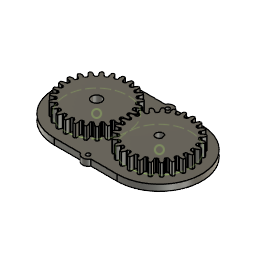
encoder gear system enclosed (Autodesk Fusion 360 design; units mm, degrees)
description: Spur Gear; Module: 2.0; Num Teeth: 25; Pressure Angle: 14.500000000000002; Backlash: 0.15 mm
Autodesk Fusion 360 part; units mm, degrees
(part 1 of 3)
sketch "Sketch1" plane through (0, 0, 0) normal (0, 0, 1) x (1, 0, 0) in component "casing bottom"
  circle A0 centre (0, 0) radius 19.5 construction
  circle A1 centre (50.4, 0) radius 15 construction
  circle A2 centre (0, 0) radius 15.5
  circle A3 centre (50.4, 0) radius 11
  circle A4 centre (13.7886, 13.7886) radius 2.2
  circle A5 centre (13.7886, 13.7886) radius 5.2
  circle A6 centre (-13.7886, 13.7886) radius 2.2
  circle A7 centre (-13.7886, 13.7886) radius 5.2
  circle A8 centre (-13.7886, -13.7886) radius 2.2
  circle A9 centre (-13.7886, -13.7886) radius 5.2
  circle A10 centre (13.7886, -13.7886) radius 2.2
  circle A11 centre (13.7886, -13.7886) radius 5.2
  line L0 (0, 0) -> (13.7886, 13.7886) construction
  line L1 (0, 0) -> (19.5, 0) construction
  circle A12 centre (35.4, 0) radius 1.7
  circle A13 centre (57.9, -12.9904) radius 1.7
  circle A14 centre (57.9, 12.9904) radius 1.7
  circle A15 centre (35.4, 0) radius 4.7
  circle A16 centre (57.9, -12.9904) radius 4.7
  circle A17 centre (57.9, 12.9904) radius 4.7
  circle A18 centre (0, 0) radius 30
  circle A19 centre (0, 0) radius 34
  line L2 (0, 0) -> (-30, 0) construction
  line L3 (50.4, 0) -> (80.4, 0) construction
  line L4 (80.4, 0) -> (84.4, 0) construction
  line L5 (-30, 0) -> (-34, 0) construction
  line L6 (0, 0) -> (50.4, 0) construction
  line L7 (25.2, 0) -> (25.2, 30) construction
  circle A20 centre (50.4, 0) radius 34
  circle A21 centre (50.4, 0) radius 30
  line L8 (0, 30) -> (50.4, 30)
  line L9 (0, 34) -> (50.4, 34)
  line L10 (0, -34) -> (50.4, -34)
  line L11 (0, -30) -> (50.4, -30)
  line L12 (25.2, 30) -> (25.2, 34) construction
  circle A22 centre (25.2, 32) radius 1.6
  circle A23 centre (25.2, 32) radius 4.6
  circle A24 centre (25.2, -32) radius 4.6
  circle A25 centre (25.2, -32) radius 1.6
  dimension "d189_1_1_1" = 39
  dimension "d190_1_1_1" = 30
  dimension "d191_1_1_1" = 50.4
  dimension "d193_1_1_1" = -4
  dimension "d195_1_1_1" = -4
  dimension "d196_1_1_1" = 4.4
  dimension "d197_1_1_1" = 3
  dimension "d199_1_1_1" = 360
  dimension "d200_1_1_1" = 45
  dimension "d201_1_1_1" = 3.4
  dimension "d209_1_1_1" = 3
  dimension "d211_1_1_1" = 360
  dimension "d243" = 60
  dimension "d245" = 4
  dimension "d261" = -4
  dimension "d264" = 3.2
  dimension "d268" = 3
  constraint coincident A0.centre A2.centre
  constraint coincident A0 A4.centre
  constraint horizontal A1.centre A0.centre
  constraint coincident A4.centre A5.centre
  constraint coincident A0 L1.end
  constraint horizontal L1
  constraint coincident A1 A12.centre
  constraint horizontal A1.centre A12.centre
  constraint coincident A19 L5.end
  constraint horizontal L2
  constraint coincident A1.centre A3.centre
  constraint parallel L2 L3
  constraint parallel L2 L4
  constraint coincident A18 L2.end
  constraint horizontal L5
  constraint midpoint L6 L7.start
  constraint perpendicular L6 L7
  constraint symmetric A18 L7 A21
  constraint symmetric A19 L7 A20
  constraint coincident A18 L8.start
  constraint coincident A21 L8.end
  constraint tangent A21 L8
  constraint tangent A18 L8
  constraint symmetric L6 L8.start L11.start
  constraint symmetric L6 L8.end L11.end
  constraint symmetric L6 L9.start L10.start
  constraint symmetric L6 L9.end L10.end
  constraint midpoint L12.end L9
  constraint coincident L8 L7.end
  constraint perpendicular L6 L12
  constraint symmetric A18 A21 L12
  constraint symmetric A19 A20 L12
  constraint midpoint L12 A22.centre
  constraint symmetric L6 A22 A25
  constraint symmetric L6 A23 A24
  measures "d189_1_1_1" diameter of A0
  measures "d190_1_1_1" diameter of A1
  measures "d191_1_1_1" distance of A0.centre A1.centre
  measures "d196_1_1_1" diameter of A4
  measures "d200_1_1_1" angle of L0 L1
  measures "d201_1_1_1" diameter of A12
  measures "d243" diameter of A18
  measures "d264" diameter of A22
extrude "Extrude5" add sketch "Sketch1" against normal blind 5 contours A2 A5 A7 A9 A11 | A2 A5 A11 A20 | A2 A5 | A2 A5 A20 | A2 A11 A20 | A2 A11 | A2 A5 A7 A9 A11 A18 A20 | A5 A20 | A5 A11 A18 A20 A21 | A11 A20 | A2 A7 | A2 A7 | A2 A9 | A2 A9 | A18 A19 A20 A21 | A18 A19 A20 L8 | A18 A19 A20 L11 | A18 A19 A20 A21 | A15 A18 A19 A21 | A18 A21 | A18 A19 L8 L11 | A19 A20 A21 L8 | A19 A20 L8 A23 | A19 A20 L11 A24 | A19 A20 A21 L11 | A3 A15 A16 A17 A19 A21 | A19 L8 L9 A23 | A20 L8 L9 A23 | A20 A21 L8 L11 | A19 L10 L11 A24 | A20 L10 L11 A24 | A12 A15 A19 | A3 A12 A15 A19 | L8 L9 A23 | L8 A23 | L11 A24 | L10 L11 A24 | L9 A23 | L10 A24 | A3 A17 | A3 A16 picked at (56.2758, 10.1772) picked at (56.2758, -10.1772) makes body 1 in component "casing bottom"
extrude "Extrude6" cut sketch "Sketch1" against normal blind 3 contours A12 A15 A19 | A3 A12 A15 A19 | A3 A17 | A3 A16 picked at (56.2758, 10.1772) picked at (56.2758, -10.1772) bodies 1 in component "casing bottom"
extrude "Extrude7" cut sketch "Sketch1" against normal blind 5 contours A2 A5 A7 A9 A11 bodies 1 in component "casing bottom"
sketch "Sketch1 (2)" plane through (0, 0, 0) normal (0, 0, 1) x (1, 0, 0) in component "casing top"
  circle A0 centre (0, 0) radius 19.5 construction
  circle A1 centre (50.4, 0) radius 15 construction
  circle A2 centre (0, 0) radius 15.5
  circle A3 centre (50.4, 0) radius 11
  circle A4 centre (13.7886, 13.7886) radius 2.2
  circle A5 centre (13.7886, 13.7886) radius 5.2
  circle A6 centre (-13.7886, 13.7886) radius 2.2
  circle A7 centre (-13.7886, 13.7886) radius 5.2
  circle A8 centre (-13.7886, -13.7886) radius 2.2
  circle A9 centre (-13.7886, -13.7886) radius 5.2
  circle A10 centre (13.7886, -13.7886) radius 2.2
  circle A11 centre (13.7886, -13.7886) radius 5.2
  line L0 (0, 0) -> (13.7886, 13.7886) construction
  line L1 (0, 0) -> (19.5, 0) construction
  circle A12 centre (35.4, 0) radius 1.7
  circle A13 centre (57.9, -12.9904) radius 1.7
  circle A14 centre (57.9, 12.9904) radius 1.7
  circle A15 centre (35.4, 0) radius 4.7
  circle A16 centre (57.9, -12.9904) radius 4.7
  circle A17 centre (57.9, 12.9904) radius 4.7
  circle A18 centre (0, 0) radius 30
  circle A19 centre (0, 0) radius 34
  line L2 (0, 0) -> (-30, 0) construction
  line L3 (50.4, 0) -> (80.4, 0) construction
  line L4 (80.4, 0) -> (84.4, 0) construction
  line L5 (-30, 0) -> (-34, 0) construction
  line L6 (0, 0) -> (50.4, 0) construction
  line L7 (25.2, 0) -> (25.2, 30) construction
  circle A20 centre (50.4, 0) radius 34
  circle A21 centre (50.4, 0) radius 30
  line L8 (0, 30) -> (50.4, 30)
  line L9 (0, 34) -> (50.4, 34)
  line L10 (0, -34) -> (50.4, -34)
  line L11 (0, -30) -> (50.4, -30)
  line L12 (25.2, 30) -> (25.2, 34) construction
  circle A22 centre (25.2, 32) radius 1.6
  circle A23 centre (25.2, 32) radius 4.6
  circle A24 centre (25.2, -32) radius 4.6
  circle A25 centre (25.2, -32) radius 1.6
  dimension "d189_1_1_1_1" = 39
  dimension "d190_1_1_1_1" = 30
  dimension "d191_1_1_1_1" = 50.4
  dimension "d193_1_1_1_1" = -4
  dimension "d195_1_1_1_1" = -4
  dimension "d196_1_1_1_1" = 4.4
  dimension "d197_1_1_1_1" = 3
  dimension "d199_1_1_1_1" = 360
  dimension "d200_1_1_1_1" = 45
  dimension "d201_1_1_1_1" = 3.4
  dimension "d209_1_1_1_1" = 3
  dimension "d211_1_1_1_1" = 360
  dimension "d243_1" = 60
  dimension "d245_1" = 4
  dimension "d261_1" = -4
  dimension "d264_1" = 3.2
  dimension "d268_1" = 3
  constraint coincident A0.centre A2.centre
  constraint coincident A0 A4.centre
  constraint horizontal A1.centre A0.centre
  constraint coincident A4.centre A5.centre
  constraint coincident A0 L1.end
  constraint horizontal L1
  constraint coincident A1 A12.centre
  constraint horizontal A1.centre A12.centre
  constraint coincident A19 L5.end
  constraint horizontal L2
  constraint coincident A1.centre A3.centre
  constraint parallel L2 L3
  constraint parallel L2 L4
  constraint coincident A18 L2.end
  constraint horizontal L5
  constraint midpoint L6 L7.start
  constraint perpendicular L6 L7
  constraint symmetric A18 L7 A21
  constraint symmetric A19 L7 A20
  constraint coincident A18 L8.start
  constraint coincident A21 L8.end
  constraint tangent A21 L8
  constraint tangent A18 L8
  constraint symmetric L6 L8.start L11.start
  constraint symmetric L6 L8.end L11.end
  constraint symmetric L6 L9.start L10.start
  constraint symmetric L6 L9.end L10.end
  constraint midpoint L12.end L9
  constraint coincident L8 L7.end
  constraint perpendicular L6 L12
  constraint symmetric A18 A21 L12
  constraint symmetric A19 A20 L12
  constraint midpoint L12 A22.centre
  constraint symmetric L6 A22 A25
  constraint symmetric L6 A23 A24
  measures "d189_1_1_1_1" diameter of A0
  measures "d190_1_1_1_1" diameter of A1
  measures "d191_1_1_1_1" distance of A0.centre A1.centre
  measures "d196_1_1_1_1" diameter of A4
  measures "d200_1_1_1_1" angle of L0 L1
  measures "d201_1_1_1_1" diameter of A12
  measures "d243_1" diameter of A18
  measures "d264_1" diameter of A22
extrude "Extrude5'" add sketch "Sketch1 (2)" against normal blind 5 separate body contours A2 A5 A7 A9 A11 | A2 A5 A11 A20 | A2 A5 | A2 A5 A20 | A2 A11 A20 | A2 A11 | A2 A5 A7 A9 A11 A18 A20 | A5 A20 | A5 A11 A18 A20 A21 | A11 A20 | A2 A7 | A2 A7 | A2 A9 | A2 A9 | A18 A19 A20 A21 | A18 A19 A20 L8 | A18 A19 A20 L11 | A18 A19 A20 A21 | A15 A18 A19 A21 | A18 A21 | A18 A19 L8 L11 | A19 A20 A21 L8 | A19 A20 L8 A23 | A19 A20 L11 A24 | A19 A20 A21 L11 | A3 A15 A16 A17 A19 A21 | A19 L8 L9 A23 | A20 L8 L9 A23 | A20 A21 L8 L11 | A19 L10 L11 A24 | A20 L10 L11 A24 | A12 A15 A19 | A3 A12 A15 A19 | L8 L9 A23 | L8 A23 | L11 A24 | L10 L11 A24 | A3 A15 | A3 A15 A16 A17 | A12 A19 | A12 A19 | L9 A23 | L10 A24 | A3 A17 | A3 A17 | A3 A16 | A3 A16 | A4 | A6 | A8 | A10 | A13 | A14 makes body 2 in component "casing top"
extrude "Extrude8" add sketch "Sketch1 (2)" along normal blind 14 contours A18 A19 L8 L11 | A19 L8 L9 A23 | A20 L8 L9 A23 | A20 A21 L8 L11 | A19 L10 L11 A24 | A20 L10 L11 A24 | L8 L9 A23 | L8 A23 | L11 A24 | L10 L11 A24 | L9 A23 | L10 A24 bodies 2 in component "casing top"
sketch "Sketch1 (3)" plane through (0, 0, 0) normal (0, 0, 1) x (1, 0, 0) in component "Spur Gear (25 teeth) motor"
  circle A0 centre (0, 0) radius 22.5492
  circle A1 centre (0, 0) radius 4.05
extrude "Extrude1" add sketch "Sketch1 (3)" along normal blind 10 separate body makes body 3 in component "Spur Gear (25 teeth) motor"
sketch "Sketch2" plane through (0, 0, 0) normal (0, 0, 1) x (1, 0, 0) in component "Spur Gear (25 teeth) motor"
  spline S0 degree 5 poles (24.1496, -1.6175) (24.1577, -1.618) (24.174, -1.6189) (24.1983, -1.6197) (24.2309, -1.6198) (24.2716, -1.6186) (24.3123, -1.6164) (24.353, -1.6135) (24.3938, -1.6103) (24.4345, -1.6069) (24.4753, -1.6032) (24.5161, -1.5993) (24.5569, -1.5949) (24.5977, -1.5901) (24.6385, -1.5848) (24.6793, -1.579) (24.7201, -1.5729) (24.7609, -1.5664) (24.8017, -1.5597) (24.8425, -1.5527) (24.8833, -1.5455) (24.9241, -1.5379) (24.9648, -1.5301) (25.0056, -1.522) (25.0464, -1.5136) (25.0871, -1.5049) (25.1279, -1.496) (25.1686, -1.4867) (25.2094, -1.4773) (25.2501, -1.4676) (25.2908, -1.4577) (25.3315, -1.4475) (25.3722, -1.4371) (25.4129, -1.4265) (25.4536, -1.4156) (25.4942, -1.4045) (25.5349, -1.3932) (25.5755, -1.3816) (25.6161, -1.3698) (25.6568, -1.3579) (25.6973, -1.3457) (25.7379, -1.3333) (25.7785, -1.3207) (25.819, -1.3079) (25.8596, -1.2949) (25.9001, -1.2816) (25.9406, -1.2682) (25.9811, -1.2546) (26.0215, -1.2408) (26.062, -1.2268) (26.1024, -1.2126) (26.1428, -1.1982) (26.1832, -1.1836) (26.2236, -1.1688) (26.2639, -1.1539) (26.3042, -1.1387) (26.3446, -1.1234) (26.3848, -1.1079) (26.4251, -1.0922) (26.4654, -1.0763) (26.5056, -1.0603) (26.5458, -1.044) (26.586, -1.0276) (26.6261, -1.0111) (26.6663, -0.9943) (26.7064, -0.9774) (26.7465, -0.9603) (26.7865, -0.943) (26.8266, -0.9256) (26.8666, -0.908) (26.9066, -0.8902) (26.9386, -0.8758) (26.9625, -0.865) (26.9785, -0.8577) (26.9865, -0.8541) knots 0 0 0 0 0 0 0.01428571 0.02857143 0.04285714 0.05714286 0.07142857 0.08571429 0.1 0.11428571 0.12857143 0.14285714 0.15714286 0.17142857 0.18571429 0.2 0.21428571 0.22857143 0.24285714 0.25714286 0.27142857 0.28571429 0.3 0.31428571 0.32857143 0.34285714 0.35714286 0.37142857 0.38571429 0.4 0.41428571 0.42857143 0.44285714 0.45714286 0.47142857 0.48571429 0.5 0.51428571 0.52857143 0.54285714 0.55714286 0.57142857 0.58571429 0.6 0.61428571 0.62857143 0.64285714 0.65714286 0.67142857 0.68571429 0.7 0.71428571 0.72857143 0.74285714 0.75714286 0.77142857 0.78571429 0.8 0.81428571 0.82857143 0.84285714 0.85714286 0.87142857 0.88571429 0.9 0.91428571 0.92857143 0.94285714 0.95714286 0.97142857 0.98571429 1 1 1 1 1 1
  spline S1 degree 5 poles (24.1496, 1.6175) (24.1577, 1.618) (24.174, 1.6189) (24.1983, 1.6197) (24.2309, 1.6198) (24.2716, 1.6186) (24.3123, 1.6164) (24.353, 1.6135) (24.3938, 1.6103) (24.4345, 1.6069) (24.4753, 1.6032) (24.5161, 1.5993) (24.5569, 1.5949) (24.5977, 1.5901) (24.6385, 1.5848) (24.6793, 1.579) (24.7201, 1.5729) (24.7609, 1.5664) (24.8017, 1.5597) (24.8425, 1.5527) (24.8833, 1.5455) (24.9241, 1.5379) (24.9648, 1.5301) (25.0056, 1.522) (25.0464, 1.5136) (25.0871, 1.5049) (25.1279, 1.496) (25.1686, 1.4867) (25.2094, 1.4773) (25.2501, 1.4676) (25.2908, 1.4577) (25.3315, 1.4475) (25.3722, 1.4371) (25.4129, 1.4265) (25.4536, 1.4156) (25.4942, 1.4045) (25.5349, 1.3932) (25.5755, 1.3816) (25.6161, 1.3698) (25.6568, 1.3579) (25.6973, 1.3457) (25.7379, 1.3333) (25.7785, 1.3207) (25.819, 1.3079) (25.8596, 1.2949) (25.9001, 1.2816) (25.9406, 1.2682) (25.9811, 1.2546) (26.0215, 1.2408) (26.062, 1.2268) (26.1024, 1.2126) (26.1428, 1.1982) (26.1832, 1.1836) (26.2236, 1.1688) (26.2639, 1.1539) (26.3042, 1.1387) (26.3446, 1.1234) (26.3848, 1.1079) (26.4251, 1.0922) (26.4654, 1.0763) (26.5056, 1.0603) (26.5458, 1.044) (26.586, 1.0276) (26.6261, 1.0111) (26.6663, 0.9943) (26.7064, 0.9774) (26.7465, 0.9603) (26.7865, 0.943) (26.8266, 0.9256) (26.8666, 0.908) (26.9066, 0.8902) (26.9386, 0.8758) (26.9625, 0.865) (26.9785, 0.8577) (26.9865, 0.8541) knots 0 0 0 0 0 0 0.01428571 0.02857143 0.04285714 0.05714286 0.07142857 0.08571429 0.1 0.11428571 0.12857143 0.14285714 0.15714286 0.17142857 0.18571429 0.2 0.21428571 0.22857143 0.24285714 0.25714286 0.27142857 0.28571429 0.3 0.31428571 0.32857143 0.34285714 0.35714286 0.37142857 0.38571429 0.4 0.41428571 0.42857143 0.44285714 0.45714286 0.47142857 0.48571429 0.5 0.51428571 0.52857143 0.54285714 0.55714286 0.57142857 0.58571429 0.6 0.61428571 0.62857143 0.64285714 0.65714286 0.67142857 0.68571429 0.7 0.71428571 0.72857143 0.74285714 0.75714286 0.77142857 0.78571429 0.8 0.81428571 0.82857143 0.84285714 0.85714286 0.87142857 0.88571429 0.9 0.91428571 0.92857143 0.94285714 0.95714286 0.97142857 0.98571429 1 1 1 1 1 1
  arc A0 (26.9865, -0.8541) -> (26.9865, 0.8541) centre (0, 0) ccw
  line L0 (22.4888, -1.5069) -> (24.1496, -1.6175)
  line L1 (22.4888, 1.5069) -> (24.1496, 1.6175)
  line L2 (22.4888, -1.5069) -> (22.4888, 1.5069)
  point P0 (24.35, -1.6137)
  point P1 (24.5514, -1.5954)
  point P2 (24.7533, -1.5676)
  point P3 (24.9557, -1.5318)
  point P4 (25.1583, -1.489)
  point P5 (25.3613, -1.4399)
  point P6 (25.5644, -1.3847)
  point P7 (25.7676, -1.324)
  point P8 (25.9709, -1.258)
  point P9 (26.1742, -1.1868)
  point P10 (26.3774, -1.1107)
  point P11 (26.5806, -1.0298)
  point P12 (26.7836, -0.9442)
  point P13 (24.35, 1.6137)
  point P14 (24.5514, 1.5954)
  point P15 (24.7533, 1.5676)
  point P16 (24.9557, 1.5318)
  point P17 (25.1583, 1.489)
  point P18 (25.3613, 1.4399)
  point P19 (25.5644, 1.3847)
  point P20 (25.7676, 1.324)
  point P21 (25.9709, 1.258)
  point P22 (26.1742, 1.1868)
  point P23 (26.3774, 1.1107)
  point P24 (26.5806, 1.0298)
  point P25 (26.7836, 0.9442)
extrude "Extrude2" add sketch "Sketch2" along normal blind 10 bodies 3 in component "Spur Gear (25 teeth) motor"
fillet "Fillet1" radius 1 2 edges at (22.4987, -1.5076, 5) (22.4987, 1.5076, 5) on bodies 3 in component "Spur Gear (25 teeth) motor"
pattern_circular "C-Pattern1" count 25 over 360 about axis through (0, 0, 0) along (0, 0, 1) of "Extrude2", "Fillet1" in component "Spur Gear (25 teeth) motor"
sketch "Sketch3" plane through (0, 0, 0) normal (0, 0, 1) x (1, 0, 0) in component "Spur Gear (25 teeth) motor"
  circle A0 centre (0, 0) radius 25 construction
sketch "Sketch1 (4)" plane through (0, 0, 0) normal (0, 0, 1) x (1, 0, 0) in component "Spur Gear (25 teeth) encoder"
  circle A0 centre (0, 0) radius 22.5492
  circle A1 centre (0, 0) radius 3.05
extrude "Extrude1'" add sketch "Sketch1 (4)" along normal blind 10 separate body makes body 4 in component "Spur Gear (25 teeth) encoder"
sketch "Sketch2 (2)" plane through (0, 0, 0) normal (0, 0, 1) x (1, 0, 0) in component "Spur Gear (25 teeth) encoder"
  spline S0 degree 5 poles (24.1496, -1.6175) (24.1577, -1.618) (24.174, -1.6189) (24.1983, -1.6197) (24.2309, -1.6198) (24.2716, -1.6186) (24.3123, -1.6164) (24.353, -1.6135) (24.3938, -1.6103) (24.4345, -1.6069) (24.4753, -1.6032) (24.5161, -1.5993) (24.5569, -1.5949) (24.5977, -1.5901) (24.6385, -1.5848) (24.6793, -1.579) (24.7201, -1.5729) (24.7609, -1.5664) (24.8017, -1.5597) (24.8425, -1.5527) (24.8833, -1.5455) (24.9241, -1.5379) (24.9648, -1.5301) (25.0056, -1.522) (25.0464, -1.5136) (25.0871, -1.5049) (25.1279, -1.496) (25.1686, -1.4867) (25.2094, -1.4773) (25.2501, -1.4676) (25.2908, -1.4577) (25.3315, -1.4475) (25.3722, -1.4371) (25.4129, -1.4265) (25.4536, -1.4156) (25.4942, -1.4045) (25.5349, -1.3932) (25.5755, -1.3816) (25.6161, -1.3698) (25.6568, -1.3579) (25.6973, -1.3457) (25.7379, -1.3333) (25.7785, -1.3207) (25.819, -1.3079) (25.8596, -1.2949) (25.9001, -1.2816) (25.9406, -1.2682) (25.9811, -1.2546) (26.0215, -1.2408) (26.062, -1.2268) (26.1024, -1.2126) (26.1428, -1.1982) (26.1832, -1.1836) (26.2236, -1.1688) (26.2639, -1.1539) (26.3042, -1.1387) (26.3446, -1.1234) (26.3848, -1.1079) (26.4251, -1.0922) (26.4654, -1.0763) (26.5056, -1.0603) (26.5458, -1.044) (26.586, -1.0276) (26.6261, -1.0111) (26.6663, -0.9943) (26.7064, -0.9774) (26.7465, -0.9603) (26.7865, -0.943) (26.8266, -0.9256) (26.8666, -0.908) (26.9066, -0.8902) (26.9386, -0.8758) (26.9625, -0.865) (26.9785, -0.8577) (26.9865, -0.8541) knots 0 0 0 0 0 0 0.01428571 0.02857143 0.04285714 0.05714286 0.07142857 0.08571429 0.1 0.11428571 0.12857143 0.14285714 0.15714286 0.17142857 0.18571429 0.2 0.21428571 0.22857143 0.24285714 0.25714286 0.27142857 0.28571429 0.3 0.31428571 0.32857143 0.34285714 0.35714286 0.37142857 0.38571429 0.4 0.41428571 0.42857143 0.44285714 0.45714286 0.47142857 0.48571429 0.5 0.51428571 0.52857143 0.54285714 0.55714286 0.57142857 0.58571429 0.6 0.61428571 0.62857143 0.64285714 0.65714286 0.67142857 0.68571429 0.7 0.71428571 0.72857143 0.74285714 0.75714286 0.77142857 0.78571429 0.8 0.81428571 0.82857143 0.84285714 0.85714286 0.87142857 0.88571429 0.9 0.91428571 0.92857143 0.94285714 0.95714286 0.97142857 0.98571429 1 1 1 1 1 1
  spline S1 degree 5 poles (24.1496, 1.6175) (24.1577, 1.618) (24.174, 1.6189) (24.1983, 1.6197) (24.2309, 1.6198) (24.2716, 1.6186) (24.3123, 1.6164) (24.353, 1.6135) (24.3938, 1.6103) (24.4345, 1.6069) (24.4753, 1.6032) (24.5161, 1.5993) (24.5569, 1.5949) (24.5977, 1.5901) (24.6385, 1.5848) (24.6793, 1.579) (24.7201, 1.5729) (24.7609, 1.5664) (24.8017, 1.5597) (24.8425, 1.5527) (24.8833, 1.5455) (24.9241, 1.5379) (24.9648, 1.5301) (25.0056, 1.522) (25.0464, 1.5136) (25.0871, 1.5049) (25.1279, 1.496) (25.1686, 1.4867) (25.2094, 1.4773) (25.2501, 1.4676) (25.2908, 1.4577) (25.3315, 1.4475) (25.3722, 1.4371) (25.4129, 1.4265) (25.4536, 1.4156) (25.4942, 1.4045) (25.5349, 1.3932) (25.5755, 1.3816) (25.6161, 1.3698) (25.6568, 1.3579) (25.6973, 1.3457) (25.7379, 1.3333) (25.7785, 1.3207) (25.819, 1.3079) (25.8596, 1.2949) (25.9001, 1.2816) (25.9406, 1.2682) (25.9811, 1.2546) (26.0215, 1.2408) (26.062, 1.2268) (26.1024, 1.2126) (26.1428, 1.1982) (26.1832, 1.1836) (26.2236, 1.1688) (26.2639, 1.1539) (26.3042, 1.1387) (26.3446, 1.1234) (26.3848, 1.1079) (26.4251, 1.0922) (26.4654, 1.0763) (26.5056, 1.0603) (26.5458, 1.044) (26.586, 1.0276) (26.6261, 1.0111) (26.6663, 0.9943) (26.7064, 0.9774) (26.7465, 0.9603) (26.7865, 0.943) (26.8266, 0.9256) (26.8666, 0.908) (26.9066, 0.8902) (26.9386, 0.8758) (26.9625, 0.865) (26.9785, 0.8577) (26.9865, 0.8541) knots 0 0 0 0 0 0 0.01428571 0.02857143 0.04285714 0.05714286 0.07142857 0.08571429 0.1 0.11428571 0.12857143 0.14285714 0.15714286 0.17142857 0.18571429 0.2 0.21428571 0.22857143 0.24285714 0.25714286 0.27142857 0.28571429 0.3 0.31428571 0.32857143 0.34285714 0.35714286 0.37142857 0.38571429 0.4 0.41428571 0.42857143 0.44285714 0.45714286 0.47142857 0.48571429 0.5 0.51428571 0.52857143 0.54285714 0.55714286 0.57142857 0.58571429 0.6 0.61428571 0.62857143 0.64285714 0.65714286 0.67142857 0.68571429 0.7 0.71428571 0.72857143 0.74285714 0.75714286 0.77142857 0.78571429 0.8 0.81428571 0.82857143 0.84285714 0.85714286 0.87142857 0.88571429 0.9 0.91428571 0.92857143 0.94285714 0.95714286 0.97142857 0.98571429 1 1 1 1 1 1
  arc A0 (26.9865, -0.8541) -> (26.9865, 0.8541) centre (0, 0) ccw
  line L0 (22.4888, -1.5069) -> (24.1496, -1.6175)
  line L1 (22.4888, 1.5069) -> (24.1496, 1.6175)
  line L2 (22.4888, -1.5069) -> (22.4888, 1.5069)
  point P0 (24.35, -1.6137)
  point P1 (24.5514, -1.5954)
  point P2 (24.7533, -1.5676)
  point P3 (24.9557, -1.5318)
  point P4 (25.1583, -1.489)
  point P5 (25.3613, -1.4399)
  point P6 (25.5644, -1.3847)
  point P7 (25.7676, -1.324)
  point P8 (25.9709, -1.258)
  point P9 (26.1742, -1.1868)
  point P10 (26.3774, -1.1107)
  point P11 (26.5806, -1.0298)
  point P12 (26.7836, -0.9442)
  point P13 (24.35, 1.6137)
  point P14 (24.5514, 1.5954)
  point P15 (24.7533, 1.5676)
  point P16 (24.9557, 1.5318)
  point P17 (25.1583, 1.489)
  point P18 (25.3613, 1.4399)
  point P19 (25.5644, 1.3847)
  point P20 (25.7676, 1.324)
  point P21 (25.9709, 1.258)
  point P22 (26.1742, 1.1868)
  point P23 (26.3774, 1.1107)
  point P24 (26.5806, 1.0298)
  point P25 (26.7836, 0.9442)
extrude "Extrude2'" add sketch "Sketch2 (2)" along normal blind 10 bodies 4 in component "Spur Gear (25 teeth) encoder"
fillet "Fillet1'" radius 1 2 edges at (22.4987, -1.5076, 5) (22.4987, 1.5076, 5) on bodies 4 in component "Spur Gear (25 teeth) encoder"
pattern_circular "C-Pattern1'" count 25 over 360 about axis through (0, 0, 0) along (0, 0, 1) of "Extrude2'", "Fillet1'" in component "Spur Gear (25 teeth) encoder"
sketch "Sketch3 (2)" plane through (0, 0, 0) normal (0, 0, 1) x (1, 0, 0) in component "Spur Gear (25 teeth) encoder"
  circle A0 centre (0, 0) radius 25 construction
sketch "Sketch4" plane through (0, 0, 0) normal (0, 0, -1) x (1, 0, 0) in component "Spur Gear (25 teeth) encoder"
  circle A0 centre (0, 0) radius 3.05
  arc A1 (21.3288, 9.9311) -> (20.8276, 8.6415) centre (21.7513, 9.0247) ccw
  line L0 (21.3288, 9.9311) -> (21.9417, 10.2168)
  spline S0 degree 5 poles (21.9417, 10.2168) (21.949, 10.2202) (21.9637, 10.2272) (21.9855, 10.2382) (22.014, 10.2538) (22.0491, 10.2745) (22.0837, 10.2961) (22.118, 10.3182) (22.1522, 10.3406) (22.1863, 10.3633) (22.2203, 10.3861) (22.2541, 10.4093) (22.2877, 10.4327) (22.3212, 10.4566) (22.3544, 10.4809) (22.3873, 10.5056) (22.4201, 10.5306) (22.4528, 10.556) (22.4853, 10.5815) (22.5177, 10.6073) (22.5499, 10.6333) (22.582, 10.6596) (22.614, 10.6861) (22.6458, 10.7128) (22.6775, 10.7398) (22.709, 10.7671) (22.7404, 10.7945) (22.7717, 10.8222) (22.8028, 10.8502) (22.8339, 10.8783) (22.8648, 10.9066) (22.8955, 10.9351) (22.9262, 10.9638) (22.9567, 10.9928) (22.9871, 11.0219) (23.0174, 11.0512) (23.0476, 11.0807) (23.0776, 11.1104) (23.1075, 11.1403) (23.1373, 11.1703) (23.167, 11.2006) (23.1966, 11.231) (23.2261, 11.2616) (23.2555, 11.2923) (23.2847, 11.3233) (23.3138, 11.3544) (23.3429, 11.3856) (23.3718, 11.4171) (23.4006, 11.4487) (23.4293, 11.4804) (23.4579, 11.5123) (23.4863, 11.5444) (23.5147, 11.5767) (23.543, 11.6091) (23.5711, 11.6416) (23.5992, 11.6743) (23.6271, 11.7072) (23.6549, 11.7402) (23.6827, 11.7733) (23.7103, 11.8066) (23.7378, 11.84) (23.7652, 11.8736) (23.7925, 11.9074) (23.8197, 11.9412) (23.8468, 11.9753) (23.8738, 12.0094) (23.9007, 12.0437) (23.9275, 12.0782) (23.9542, 12.1127) (23.9808, 12.1474) (24.0073, 12.1823) (24.0284, 12.2103) (24.0442, 12.2313) (24.0547, 12.2454) (24.0599, 12.2524) knots 0 0 0 0 0 0 0.01428571 0.02857143 0.04285714 0.05714286 0.07142857 0.08571429 0.1 0.11428571 0.12857143 0.14285714 0.15714286 0.17142857 0.18571429 0.2 0.21428571 0.22857143 0.24285714 0.25714286 0.27142857 0.28571429 0.3 0.31428571 0.32857143 0.34285714 0.35714286 0.37142857 0.38571429 0.4 0.41428571 0.42857143 0.44285714 0.45714286 0.47142857 0.48571429 0.5 0.51428571 0.52857143 0.54285714 0.55714286 0.57142857 0.58571429 0.6 0.61428571 0.62857143 0.64285714 0.65714286 0.67142857 0.68571429 0.7 0.71428571 0.72857143 0.74285714 0.75714286 0.77142857 0.78571429 0.8 0.81428571 0.82857143 0.84285714 0.85714286 0.87142857 0.88571429 0.9 0.91428571 0.92857143 0.94285714 0.95714286 0.97142857 0.98571429 1 1 1 1 1 1
  arc A2 (24.0599, 12.2524) -> (23.237, 13.7493) centre (0, 0) ccw
  spline S1 degree 5 poles (20.3832, 13.0515) (20.3901, 13.0559) (20.4039, 13.0645) (20.4248, 13.077) (20.4533, 13.0928) (20.4895, 13.1113) (20.5263, 13.129) (20.5634, 13.1461) (20.6006, 13.1629) (20.638, 13.1796) (20.6755, 13.196) (20.7132, 13.2122) (20.751, 13.228) (20.7891, 13.2435) (20.8274, 13.2585) (20.8659, 13.2731) (20.9046, 13.2873) (20.9435, 13.3013) (20.9825, 13.3151) (21.0216, 13.3286) (21.0609, 13.3419) (21.1002, 13.3549) (21.1397, 13.3677) (21.1794, 13.3803) (21.2191, 13.3926) (21.259, 13.4046) (21.2991, 13.4164) (21.3392, 13.4279) (21.3795, 13.4393) (21.4198, 13.4504) (21.4603, 13.4613) (21.5009, 13.472) (21.5415, 13.4825) (21.5823, 13.4928) (21.6232, 13.5028) (21.6642, 13.5127) (21.7052, 13.5224) (21.7464, 13.5318) (21.7877, 13.5411) (21.829, 13.5501) (21.8705, 13.559) (21.912, 13.5677) (21.9536, 13.5762) (21.9953, 13.5845) (22.0371, 13.5926) (22.079, 13.6006) (22.1209, 13.6083) (22.163, 13.6159) (22.2051, 13.6233) (22.2473, 13.6305) (22.2895, 13.6375) (22.3319, 13.6444) (22.3743, 13.651) (22.4168, 13.6575) (22.4594, 13.6639) (22.502, 13.67) (22.5447, 13.676) (22.5875, 13.6818) (22.6303, 13.6875) (22.6733, 13.693) (22.7162, 13.6983) (22.7593, 13.7034) (22.8024, 13.7084) (22.8456, 13.7132) (22.8888, 13.7179) (22.9321, 13.7224) (22.9755, 13.7267) (23.0189, 13.7309) (23.0624, 13.7349) (23.106, 13.7387) (23.1496, 13.7424) (23.1845, 13.7452) (23.2107, 13.7473) (23.2282, 13.7486) (23.237, 13.7493) knots 0 0 0 0 0 0 0.01428571 0.02857143 0.04285714 0.05714286 0.07142857 0.08571429 0.1 0.11428571 0.12857143 0.14285714 0.15714286 0.17142857 0.18571429 0.2 0.21428571 0.22857143 0.24285714 0.25714286 0.27142857 0.28571429 0.3 0.31428571 0.32857143 0.34285714 0.35714286 0.37142857 0.38571429 0.4 0.41428571 0.42857143 0.44285714 0.45714286 0.47142857 0.48571429 0.5 0.51428571 0.52857143 0.54285714 0.55714286 0.57142857 0.58571429 0.6 0.61428571 0.62857143 0.64285714 0.65714286 0.67142857 0.68571429 0.7 0.71428571 0.72857143 0.74285714 0.75714286 0.77142857 0.78571429 0.8 0.81428571 0.82857143 0.84285714 0.85714286 0.87142857 0.88571429 0.9 0.91428571 0.92857143 0.94285714 0.95714286 0.97142857 0.98571429 1 1 1 1 1 1
  line L1 (20.3832, 13.0515) -> (19.8137, 12.6872)
  arc A3 (18.4563, 12.955) -> (19.8137, 12.6872) centre (19.2748, 13.5295) ccw
  arc A4 (18.4563, 12.955) -> (18.0243, 13.5496) centre (0, 0) ccw
  arc A5 (18.189, 14.9234) -> (18.0243, 13.5496) centre (18.8236, 14.1505) ccw
  line L2 (18.189, 14.9234) -> (18.7115, 15.3525)
  spline S2 degree 5 poles (18.7115, 15.3525) (18.7178, 15.3576) (18.7303, 15.3681) (18.7486, 15.3842) (18.7724, 15.4063) (18.8012, 15.4351) (18.8294, 15.4646) (18.8571, 15.4946) (18.8846, 15.5248) (18.912, 15.5552) (18.9392, 15.5858) (18.9663, 15.6166) (18.993, 15.6477) (19.0195, 15.6791) (19.0456, 15.7109) (19.0714, 15.7431) (19.0969, 15.7755) (19.1222, 15.8081) (19.1473, 15.8409) (19.1723, 15.874) (19.1971, 15.9072) (19.2216, 15.9406) (19.246, 15.9742) (19.2702, 16.008) (19.2942, 16.0421) (19.3179, 16.0763) (19.3415, 16.1107) (19.3649, 16.1453) (19.3881, 16.1801) (19.4112, 16.2151) (19.4341, 16.2502) (19.4568, 16.2854) (19.4793, 16.3209) (19.5017, 16.3565) (19.5239, 16.3923) (19.5459, 16.4282) (19.5678, 16.4643) (19.5895, 16.5005) (19.6111, 16.5369) (19.6325, 16.5734) (19.6537, 16.6101) (19.6748, 16.6469) (19.6958, 16.6839) (19.7166, 16.721) (19.7372, 16.7582) (19.7577, 16.7956) (19.778, 16.8331) (19.7982, 16.8707) (19.8182, 16.9085) (19.8381, 16.9464) (19.8579, 16.9844) (19.8775, 17.0225) (19.8969, 17.0608) (19.9163, 17.0992) (19.9354, 17.1378) (19.9545, 17.1764) (19.9734, 17.2152) (19.9921, 17.2541) (20.0107, 17.2931) (20.0292, 17.3322) (20.0475, 17.3714) (20.0657, 17.4108) (20.0838, 17.4502) (20.1017, 17.4898) (20.1195, 17.5295) (20.1372, 17.5693) (20.1547, 17.6092) (20.1721, 17.6492) (20.1893, 17.6893) (20.2064, 17.7296) (20.2234, 17.7699) (20.2369, 17.8023) (20.247, 17.8266) (20.2536, 17.8428) (20.257, 17.8509) knots 0 0 0 0 0 0 0.01428571 0.02857143 0.04285714 0.05714286 0.07142857 0.08571429 0.1 0.11428571 0.12857143 0.14285714 0.15714286 0.17142857 0.18571429 0.2 0.21428571 0.22857143 0.24285714 0.25714286 0.27142857 0.28571429 0.3 0.31428571 0.32857143 0.34285714 0.35714286 0.37142857 0.38571429 0.4 0.41428571 0.42857143 0.44285714 0.45714286 0.47142857 0.48571429 0.5 0.51428571 0.52857143 0.54285714 0.55714286 0.57142857 0.58571429 0.6 0.61428571 0.62857143 0.64285714 0.65714286 0.67142857 0.68571429 0.7 0.71428571 0.72857143 0.74285714 0.75714286 0.77142857 0.78571429 0.8 0.81428571 0.82857143 0.84285714 0.85714286 0.87142857 0.88571429 0.9 0.91428571 0.92857143 0.94285714 0.95714286 0.97142857 0.98571429 1 1 1 1 1 1
  arc A6 (20.257, 17.8509) -> (19.0876, 19.0961) centre (0, 0) ccw
  spline S3 degree 5 poles (16.4971, 17.7106) (16.5026, 17.7166) (16.5138, 17.7283) (16.531, 17.7456) (16.5547, 17.768) (16.5852, 17.7949) (16.6164, 17.8212) (16.648, 17.847) (16.6799, 17.8726) (16.712, 17.898) (16.7442, 17.9232) (16.7767, 17.9483) (16.8094, 17.973) (16.8424, 17.9974) (16.8758, 18.0215) (16.9095, 18.0452) (16.9434, 18.0687) (16.9776, 18.0919) (17.012, 18.1149) (17.0465, 18.1377) (17.0812, 18.1604) (17.1161, 18.1828) (17.1512, 18.205) (17.1864, 18.227) (17.2219, 18.2488) (17.2576, 18.2704) (17.2934, 18.2917) (17.3294, 18.3129) (17.3656, 18.3339) (17.4019, 18.3547) (17.4384, 18.3753) (17.475, 18.3958) (17.5118, 18.4161) (17.5487, 18.4362) (17.5858, 18.4561) (17.6231, 18.4758) (17.6605, 18.4954) (17.698, 18.5148) (17.7356, 18.534) (17.7734, 18.5531) (17.8114, 18.572) (17.8494, 18.5907) (17.8876, 18.6093) (17.926, 18.6277) (17.9644, 18.646) (18.003, 18.6641) (18.0417, 18.682) (18.0805, 18.6998) (18.1195, 18.7174) (18.1586, 18.7349) (18.1978, 18.7522) (18.2371, 18.7694) (18.2765, 18.7864) (18.316, 18.8033) (18.3557, 18.82) (18.3955, 18.8366) (18.4353, 18.853) (18.4753, 18.8693) (18.5154, 18.8854) (18.5556, 18.9014) (18.5959, 18.9172) (18.6364, 18.9329) (18.6769, 18.9485) (18.7175, 18.9639) (18.7582, 18.9791) (18.7991, 18.9942) (18.84, 19.0092) (18.881, 19.0241) (18.9221, 19.0388) (18.9634, 19.0533) (19.0047, 19.0677) (19.0378, 19.0792) (19.0627, 19.0877) (19.0793, 19.0933) (19.0876, 19.0961) knots 0 0 0 0 0 0 0.01428571 0.02857143 0.04285714 0.05714286 0.07142857 0.08571429 0.1 0.11428571 0.12857143 0.14285714 0.15714286 0.17142857 0.18571429 0.2 0.21428571 0.22857143 0.24285714 0.25714286 0.27142857 0.28571429 0.3 0.31428571 0.32857143 0.34285714 0.35714286 0.37142857 0.38571429 0.4 0.41428571 0.42857143 0.44285714 0.45714286 0.47142857 0.48571429 0.5 0.51428571 0.52857143 0.54285714 0.55714286 0.57142857 0.58571429 0.6 0.61428571 0.62857143 0.64285714 0.65714286 0.67142857 0.68571429 0.7 0.71428571 0.72857143 0.74285714 0.75714286 0.77142857 0.78571429 0.8 0.81428571 0.82857143 0.84285714 0.85714286 0.87142857 0.88571429 0.9 0.91428571 0.92857143 0.94285714 0.95714286 0.97142857 0.98571429 1 1 1 1 1 1
  line L3 (16.4971, 17.7106) -> (16.036, 17.216)
  arc A7 (14.6547, 17.1379) -> (16.036, 17.216) centre (15.3046, 17.8979) ccw
  arc A8 (14.6547, 17.1379) -> (14.0883, 17.6064) centre (0, 0) ccw
  arc A9 (13.9062, 18.9779) -> (14.0883, 17.6064) centre (14.7131, 18.3872) ccw
  line L4 (13.9062, 18.9779) -> (14.3057, 19.5235)
  spline S4 degree 5 poles (14.3057, 19.5235) (14.3105, 19.5301) (14.3199, 19.5433) (14.3337, 19.5634) (14.3512, 19.5908) (14.372, 19.6259) (14.3919, 19.6614) (14.4113, 19.6974) (14.4305, 19.7335) (14.4494, 19.7697) (14.4682, 19.8061) (14.4867, 19.8427) (14.5049, 19.8795) (14.5227, 19.9165) (14.5401, 19.9538) (14.5571, 19.9913) (14.5737, 20.0291) (14.5901, 20.067) (14.6063, 20.105) (14.6223, 20.1432) (14.638, 20.1815) (14.6535, 20.22) (14.6687, 20.2586) (14.6837, 20.2974) (14.6985, 20.3363) (14.713, 20.3754) (14.7273, 20.4146) (14.7413, 20.454) (14.7552, 20.4934) (14.7688, 20.533) (14.7822, 20.5727) (14.7955, 20.6125) (14.8085, 20.6524) (14.8213, 20.6925) (14.8339, 20.7327) (14.8463, 20.7729) (14.8586, 20.8133) (14.8706, 20.8538) (14.8824, 20.8944) (14.8941, 20.9351) (14.9055, 20.9759) (14.9168, 21.0168) (14.9279, 21.0578) (14.9388, 21.0989) (14.9495, 21.1401) (14.9601, 21.1814) (14.9704, 21.2228) (14.9806, 21.2643) (14.9907, 21.3059) (15.0005, 21.3475) (15.0102, 21.3893) (15.0197, 21.4311) (15.029, 21.473) (15.0382, 21.515) (15.0471, 21.5571) (15.056, 21.5993) (15.0646, 21.6415) (15.0731, 21.6838) (15.0814, 21.7262) (15.0896, 21.7687) (15.0976, 21.8113) (15.1055, 21.8539) (15.1131, 21.8966) (15.1207, 21.9394) (15.128, 21.9823) (15.1352, 22.0252) (15.1423, 22.0683) (15.1491, 22.1113) (15.1559, 22.1545) (15.1625, 22.1977) (15.1689, 22.241) (15.1739, 22.2757) (15.1776, 22.3017) (15.18, 22.3191) (15.1812, 22.3278) knots 0 0 0 0 0 0 0.01428571 0.02857143 0.04285714 0.05714286 0.07142857 0.08571429 0.1 0.11428571 0.12857143 0.14285714 0.15714286 0.17142857 0.18571429 0.2 0.21428571 0.22857143 0.24285714 0.25714286 0.27142857 0.28571429 0.3 0.31428571 0.32857143 0.34285714 0.35714286 0.37142857 0.38571429 0.4 0.41428571 0.42857143 0.44285714 0.45714286 0.47142857 0.48571429 0.5 0.51428571 0.52857143 0.54285714 0.55714286 0.57142857 0.58571429 0.6 0.61428571 0.62857143 0.64285714 0.65714286 0.67142857 0.68571429 0.7 0.71428571 0.72857143 0.74285714 0.75714286 0.77142857 0.78571429 0.8 0.81428571 0.82857143 0.84285714 0.85714286 0.87142857 0.88571429 0.9 0.91428571 0.92857143 0.94285714 0.95714286 0.97142857 0.98571429 1 1 1 1 1 1
  arc A10 (15.1812, 22.3278) -> (13.739, 23.2431) centre (0, 0) ccw
  spline S5 degree 5 poles (11.5743, 21.2568) (11.5782, 21.264) (11.5862, 21.2782) (11.5985, 21.2992) (11.6159, 21.3267) (11.6387, 21.3604) (11.6624, 21.3936) (11.6867, 21.4265) (11.7112, 21.4592) (11.7359, 21.4918) (11.7609, 21.5243) (11.7861, 21.5566) (11.8116, 21.5887) (11.8375, 21.6205) (11.8639, 21.6521) (11.8906, 21.6835) (11.9176, 21.7147) (11.945, 21.7457) (11.9725, 21.7765) (12.0003, 21.8072) (12.0283, 21.8377) (12.0565, 21.8681) (12.0849, 21.8984) (12.1136, 21.9285) (12.1426, 21.9584) (12.1717, 21.9881) (12.2011, 22.0178) (12.2307, 22.0472) (12.2605, 22.0766) (12.2906, 22.1057) (12.3208, 22.1348) (12.3512, 22.1637) (12.3817, 22.1925) (12.4125, 22.2212) (12.4435, 22.2497) (12.4747, 22.2781) (12.506, 22.3063) (12.5375, 22.3344) (12.5692, 22.3624) (12.6011, 22.3903) (12.6331, 22.418) (12.6653, 22.4457) (12.6977, 22.4732) (12.7303, 22.5005) (12.763, 22.5278) (12.7958, 22.5549) (12.8289, 22.5819) (12.8621, 22.6088) (12.8954, 22.6355) (12.9289, 22.6622) (12.9626, 22.6887) (12.9964, 22.7151) (13.0303, 22.7414) (13.0644, 22.7676) (13.0987, 22.7936) (13.1331, 22.8196) (13.1676, 22.8454) (13.2023, 22.8711) (13.2371, 22.8967) (13.2721, 22.9222) (13.3072, 22.9475) (13.3424, 22.9728) (13.3778, 22.9979) (13.4133, 23.0229) (13.449, 23.0478) (13.4848, 23.0726) (13.5207, 23.0973) (13.5567, 23.1219) (13.5929, 23.1464) (13.6292, 23.1707) (13.6657, 23.195) (13.6949, 23.2143) (13.7169, 23.2287) (13.7316, 23.2383) (13.739, 23.2431) knots 0 0 0 0 0 0 0.01428571 0.02857143 0.04285714 0.05714286 0.07142857 0.08571429 0.1 0.11428571 0.12857143 0.14285714 0.15714286 0.17142857 0.18571429 0.2 0.21428571 0.22857143 0.24285714 0.25714286 0.27142857 0.28571429 0.3 0.31428571 0.32857143 0.34285714 0.35714286 0.37142857 0.38571429 0.4 0.41428571 0.42857143 0.44285714 0.45714286 0.47142857 0.48571429 0.5 0.51428571 0.52857143 0.54285714 0.55714286 0.57142857 0.58571429 0.6 0.61428571 0.62857143 0.64285714 0.65714286 0.67142857 0.68571429 0.7 0.71428571 0.72857143 0.74285714 0.75714286 0.77142857 0.78571429 0.8 0.81428571 0.82857143 0.84285714 0.85714286 0.87142857 0.88571429 0.9 0.91428571 0.92857143 0.94285714 0.95714286 0.97142857 0.98571429 1 1 1 1 1 1
  line L5 (11.5743, 21.2568) -> (11.2508, 20.6632)
  arc A11 (9.9322, 20.2439) -> (11.2508, 20.6632) centre (10.3727, 21.1417) ccw
  arc A12 (9.9322, 20.2439) -> (9.2672, 20.5569) centre (0, 0) ccw
  arc A13 (8.7497, 21.84) -> (9.2672, 20.5569) centre (9.6782, 21.4685) ccw
  line L6 (8.7497, 21.84) -> (9.0009, 22.4678)
  spline S6 degree 5 poles (9.0009, 22.4678) (9.0039, 22.4754) (9.0098, 22.4905) (9.0182, 22.5135) (9.0283, 22.5444) (9.0397, 22.5834) (9.0502, 22.6229) (9.06, 22.6625) (9.0696, 22.7022) (9.0789, 22.7421) (9.0881, 22.782) (9.0969, 22.822) (9.1054, 22.8621) (9.1134, 22.9024) (9.1209, 22.9429) (9.1281, 22.9835) (9.1349, 23.0241) (9.1413, 23.0649) (9.1475, 23.1058) (9.1535, 23.1468) (9.1592, 23.1878) (9.1646, 23.2289) (9.1698, 23.2701) (9.1747, 23.3114) (9.1793, 23.3528) (9.1836, 23.3942) (9.1877, 23.4358) (9.1915, 23.4774) (9.1951, 23.519) (9.1985, 23.5608) (9.2016, 23.6026) (9.2045, 23.6444) (9.2072, 23.6863) (9.2097, 23.7283) (9.2119, 23.7704) (9.2139, 23.8125) (9.2157, 23.8546) (9.2173, 23.8968) (9.2186, 23.9391) (9.2198, 23.9814) (9.2207, 24.0238) (9.2215, 24.0662) (9.222, 24.1087) (9.2224, 24.1512) (9.2225, 24.1938) (9.2225, 24.2364) (9.2222, 24.2791) (9.2218, 24.3218) (9.2211, 24.3645) (9.2203, 24.4073) (9.2193, 24.4501) (9.2181, 24.493) (9.2167, 24.5359) (9.2151, 24.5789) (9.2134, 24.6219) (9.2114, 24.6649) (9.2093, 24.708) (9.207, 24.7511) (9.2045, 24.7943) (9.2019, 24.8375) (9.199, 24.8807) (9.196, 24.9239) (9.1929, 24.9672) (9.1895, 25.0105) (9.186, 25.0539) (9.1823, 25.0973) (9.1784, 25.1407) (9.1743, 25.1841) (9.1701, 25.2276) (9.1658, 25.2711) (9.1612, 25.3146) (9.1574, 25.3494) (9.1545, 25.3756) (9.1526, 25.393) (9.1516, 25.4017) knots 0 0 0 0 0 0 0.01428571 0.02857143 0.04285714 0.05714286 0.07142857 0.08571429 0.1 0.11428571 0.12857143 0.14285714 0.15714286 0.17142857 0.18571429 0.2 0.21428571 0.22857143 0.24285714 0.25714286 0.27142857 0.28571429 0.3 0.31428571 0.32857143 0.34285714 0.35714286 0.37142857 0.38571429 0.4 0.41428571 0.42857143 0.44285714 0.45714286 0.47142857 0.48571429 0.5 0.51428571 0.52857143 0.54285714 0.55714286 0.57142857 0.58571429 0.6 0.61428571 0.62857143 0.64285714 0.65714286 0.67142857 0.68571429 0.7 0.71428571 0.72857143 0.74285714 0.75714286 0.77142857 0.78571429 0.8 0.81428571 0.82857143 0.84285714 0.85714286 0.87142857 0.88571429 0.9 0.91428571 0.92857143 0.94285714 0.95714286 0.97142857 0.98571429 1 1 1 1 1 1
  arc A14 (9.1516, 25.4017) -> (7.527, 25.9296) centre (0, 0) ccw
  spline S7 degree 5 poles (5.9243, 23.4674) (5.9263, 23.4753) (5.9305, 23.4911) (5.9372, 23.5145) (5.9472, 23.5455) (5.9609, 23.5838) (5.9756, 23.6218) (5.9909, 23.6597) (6.0066, 23.6975) (6.0224, 23.7352) (6.0385, 23.7728) (6.0549, 23.8104) (6.0716, 23.8479) (6.0888, 23.8852) (6.1065, 23.9223) (6.1246, 23.9594) (6.143, 23.9963) (6.1618, 24.0331) (6.1808, 24.0698) (6.2, 24.1064) (6.2195, 24.143) (6.2393, 24.1794) (6.2593, 24.2158) (6.2797, 24.2521) (6.3002, 24.2882) (6.3211, 24.3243) (6.3422, 24.3603) (6.3636, 24.3962) (6.3851, 24.432) (6.4069, 24.4678) (6.429, 24.5034) (6.4512, 24.539) (6.4737, 24.5745) (6.4964, 24.6099) (6.5193, 24.6452) (6.5424, 24.6805) (6.5657, 24.7156) (6.5893, 24.7507) (6.613, 24.7857) (6.637, 24.8206) (6.6611, 24.8555) (6.6854, 24.8902) (6.7099, 24.9249) (6.7347, 24.9595) (6.7596, 24.994) (6.7847, 25.0285) (6.8099, 25.0629) (6.8354, 25.0971) (6.861, 25.1314) (6.8869, 25.1655) (6.9129, 25.1996) (6.939, 25.2335) (6.9654, 25.2674) (6.9919, 25.3013) (7.0186, 25.335) (7.0455, 25.3687) (7.0725, 25.4023) (7.0997, 25.4358) (7.1271, 25.4693) (7.1546, 25.5027) (7.1823, 25.5359) (7.2102, 25.5692) (7.2382, 25.6023) (7.2664, 25.6354) (7.2947, 25.6684) (7.3232, 25.7013) (7.3518, 25.7341) (7.3806, 25.7669) (7.4096, 25.7996) (7.4387, 25.8322) (7.468, 25.8648) (7.4915, 25.8907) (7.5092, 25.9102) (7.5211, 25.9231) (7.527, 25.9296) knots 0 0 0 0 0 0 0.01428571 0.02857143 0.04285714 0.05714286 0.07142857 0.08571429 0.1 0.11428571 0.12857143 0.14285714 0.15714286 0.17142857 0.18571429 0.2 0.21428571 0.22857143 0.24285714 0.25714286 0.27142857 0.28571429 0.3 0.31428571 0.32857143 0.34285714 0.35714286 0.37142857 0.38571429 0.4 0.41428571 0.42857143 0.44285714 0.45714286 0.47142857 0.48571429 0.5 0.51428571 0.52857143 0.54285714 0.55714286 0.57142857 0.58571429 0.6 0.61428571 0.62857143 0.64285714 0.65714286 0.67142857 0.68571429 0.7 0.71428571 0.72857143 0.74285714 0.75714286 0.77142857 0.78571429 0.8 0.81428571 0.82857143 0.84285714 0.85714286 0.87142857 0.88571429 0.9 0.91428571 0.92857143 0.94285714 0.95714286 0.97142857 0.98571429 1 1 1 1 1 1
  line L7 (5.9243, 23.4674) -> (5.7586, 22.8119)
  arc A15 (4.5857, 22.078) -> (5.7586, 22.8119) centre (4.7891, 23.0571) ccw
  arc A16 (4.5857, 22.078) -> (3.8637, 22.2157) centre (0, 0) ccw
  arc A17 (3.0434, 23.3299) -> (3.8637, 22.2157) centre (4.0351, 23.2009) ccw
  line L8 (3.0434, 23.3299) -> (3.1306, 24.0004)
  spline S8 degree 5 poles (3.1306, 24.0004) (3.1317, 24.0084) (3.1336, 24.0246) (3.136, 24.0489) (3.1381, 24.0813) (3.1394, 24.122) (3.1398, 24.1628) (3.1395, 24.2036) (3.1388, 24.2445) (3.138, 24.2854) (3.1369, 24.3264) (3.1355, 24.3673) (3.1337, 24.4083) (3.1315, 24.4493) (3.1287, 24.4904) (3.1256, 24.5314) (3.122, 24.5725) (3.1181, 24.6137) (3.1139, 24.6548) (3.1095, 24.696) (3.1048, 24.7371) (3.0999, 24.7783) (3.0946, 24.8195) (3.0891, 24.8607) (3.0833, 24.9019) (3.0772, 24.9431) (3.0708, 24.9844) (3.0642, 25.0256) (3.0573, 25.0669) (3.0502, 25.1081) (3.0428, 25.1494) (3.0352, 25.1907) (3.0274, 25.2319) (3.0193, 25.2732) (3.011, 25.3145) (3.0025, 25.3557) (2.9938, 25.397) (2.9848, 25.4383) (2.9756, 25.4796) (2.9662, 25.5209) (2.9566, 25.5621) (2.9468, 25.6034) (2.9367, 25.6447) (2.9265, 25.686) (2.916, 25.7272) (2.9054, 25.7685) (2.8945, 25.8098) (2.8835, 25.851) (2.8722, 25.8923) (2.8608, 25.9335) (2.8492, 25.9747) (2.8373, 26.016) (2.8253, 26.0572) (2.8131, 26.0984) (2.8007, 26.1396) (2.7881, 26.1808) (2.7754, 26.222) (2.7624, 26.2632) (2.7493, 26.3044) (2.736, 26.3456) (2.7225, 26.3867) (2.7088, 26.4279) (2.695, 26.469) (2.6809, 26.5101) (2.6667, 26.5512) (2.6523, 26.5923) (2.6378, 26.6334) (2.6231, 26.6745) (2.6082, 26.7155) (2.5931, 26.7566) (2.5779, 26.7976) (2.5656, 26.8304) (2.5563, 26.855) (2.55, 26.8714) (2.5469, 26.8796) knots 0 0 0 0 0 0 0.01428571 0.02857143 0.04285714 0.05714286 0.07142857 0.08571429 0.1 0.11428571 0.12857143 0.14285714 0.15714286 0.17142857 0.18571429 0.2 0.21428571 0.22857143 0.24285714 0.25714286 0.27142857 0.28571429 0.3 0.31428571 0.32857143 0.34285714 0.35714286 0.37142857 0.38571429 0.4 0.41428571 0.42857143 0.44285714 0.45714286 0.47142857 0.48571429 0.5 0.51428571 0.52857143 0.54285714 0.55714286 0.57142857 0.58571429 0.6 0.61428571 0.62857143 0.64285714 0.65714286 0.67142857 0.68571429 0.7 0.71428571 0.72857143 0.74285714 0.75714286 0.77142857 0.78571429 0.8 0.81428571 0.82857143 0.84285714 0.85714286 0.87142857 0.88571429 0.9 0.91428571 0.92857143 0.94285714 0.95714286 0.97142857 0.98571429 1 1 1 1 1 1
  arc A18 (2.5469, 26.8796) -> (0.8421, 26.9869) centre (0, 0) ccw
  spline S9 degree 5 poles (-0.0979, 24.2035) (-0.0979, 24.2116) (-0.0978, 24.2279) (-0.0971, 24.2523) (-0.0952, 24.2848) (-0.0914, 24.3253) (-0.0866, 24.3658) (-0.0812, 24.4063) (-0.0755, 24.4467) (-0.0695, 24.4872) (-0.0633, 24.5277) (-0.0568, 24.5682) (-0.0498, 24.6086) (-0.0425, 24.649) (-0.0346, 24.6894) (-0.0263, 24.7297) (-0.0176, 24.7701) (-0.0086, 24.8104) (0.0007, 24.8507) (0.0102, 24.891) (0.02, 24.9312) (0.0301, 24.9714) (0.0405, 25.0117) (0.0511, 25.0518) (0.0621, 25.092) (0.0733, 25.1321) (0.0848, 25.1722) (0.0965, 25.2123) (0.1085, 25.2524) (0.1208, 25.2924) (0.1332, 25.3324) (0.1459, 25.3724) (0.1589, 25.4124) (0.172, 25.4523) (0.1855, 25.4922) (0.1991, 25.5321) (0.2129, 25.572) (0.227, 25.6118) (0.2413, 25.6516) (0.2558, 25.6914) (0.2705, 25.7311) (0.2854, 25.7709) (0.3006, 25.8105) (0.3159, 25.8502) (0.3314, 25.8898) (0.3472, 25.9294) (0.3631, 25.969) (0.3792, 26.0086) (0.3956, 26.0481) (0.4121, 26.0876) (0.4288, 26.127) (0.4457, 26.1664) (0.4628, 26.2058) (0.4801, 26.2452) (0.4975, 26.2845) (0.5152, 26.3238) (0.533, 26.3631) (0.551, 26.4023) (0.5692, 26.4415) (0.5876, 26.4807) (0.6061, 26.5199) (0.6248, 26.559) (0.6437, 26.598) (0.6628, 26.6371) (0.6821, 26.6761) (0.7015, 26.715) (0.721, 26.754) (0.7408, 26.7929) (0.7607, 26.8318) (0.7808, 26.8706) (0.8011, 26.9094) (0.8174, 26.9404) (0.8297, 26.9636) (0.838, 26.9791) (0.8421, 26.9869) knots 0 0 0 0 0 0 0.01428571 0.02857143 0.04285714 0.05714286 0.07142857 0.08571429 0.1 0.11428571 0.12857143 0.14285714 0.15714286 0.17142857 0.18571429 0.2 0.21428571 0.22857143 0.24285714 0.25714286 0.27142857 0.28571429 0.3 0.31428571 0.32857143 0.34285714 0.35714286 0.37142857 0.38571429 0.4 0.41428571 0.42857143 0.44285714 0.45714286 0.47142857 0.48571429 0.5 0.51428571 0.52857143 0.54285714 0.55714286 0.57142857 0.58571429 0.6 0.61428571 0.62857143 0.64285714 0.65714286 0.67142857 0.68571429 0.7 0.71428571 0.72857143 0.74285714 0.75714286 0.77142857 0.78571429 0.8 0.81428571 0.82857143 0.84285714 0.85714286 0.87142857 0.88571429 0.9 0.91428571 0.92857143 0.94285714 0.95714286 0.97142857 0.98571429 1 1 1 1 1 1
  line L9 (-0.0979, 24.2035) -> (-0.0954, 23.5274)
  arc A19 (-1.0489, 22.5248) -> (-0.0954, 23.5274) centre (-1.0954, 23.5237) ccw
  arc A20 (-1.0489, 22.5248) -> (-1.7825, 22.4786) centre (0, 0) ccw
  arc A21 (-2.8541, 23.3538) -> (-1.7825, 22.4786) centre (-1.8615, 23.4755) ccw
  line L10 (-2.8541, 23.3538) -> (-2.9364, 24.0249)
  spline S10 degree 5 poles (-2.9364, 24.0249) (-2.9374, 24.033) (-2.9395, 24.0491) (-2.9433, 24.0732) (-2.9493, 24.1052) (-2.9581, 24.1449) (-2.9679, 24.1845) (-2.9784, 24.224) (-2.9891, 24.2634) (-3.0001, 24.3028) (-3.0114, 24.3422) (-3.0229, 24.3815) (-3.0348, 24.4208) (-3.0472, 24.46) (-3.0601, 24.499) (-3.0734, 24.538) (-3.087, 24.577) (-3.101, 24.6158) (-3.1153, 24.6546) (-3.1298, 24.6934) (-3.1446, 24.7321) (-3.1596, 24.7708) (-3.1749, 24.8094) (-3.1905, 24.8479) (-3.2064, 24.8864) (-3.2226, 24.9248) (-3.239, 24.9631) (-3.2557, 25.0014) (-3.2726, 25.0397) (-3.2898, 25.0779) (-3.3072, 25.116) (-3.3248, 25.1541) (-3.3426, 25.1921) (-3.3607, 25.2301) (-3.379, 25.268) (-3.3975, 25.3058) (-3.4163, 25.3437) (-3.4352, 25.3814) (-3.4544, 25.4191) (-3.4738, 25.4567) (-3.4934, 25.4943) (-3.5131, 25.5319) (-3.5331, 25.5694) (-3.5533, 25.6068) (-3.5737, 25.6442) (-3.5943, 25.6815) (-3.615, 25.7187) (-3.636, 25.756) (-3.6571, 25.7931) (-3.6785, 25.8302) (-3.7, 25.8673) (-3.7217, 25.9043) (-3.7436, 25.9412) (-3.7657, 25.9781) (-3.7879, 26.0149) (-3.8104, 26.0517) (-3.833, 26.0884) (-3.8558, 26.1251) (-3.8787, 26.1617) (-3.9019, 26.1983) (-3.9252, 26.2348) (-3.9486, 26.2712) (-3.9723, 26.3076) (-3.9961, 26.344) (-4.0201, 26.3802) (-4.0442, 26.4165) (-4.0685, 26.4527) (-4.093, 26.4888) (-4.1176, 26.5248) (-4.1424, 26.5608) (-4.1674, 26.5968) (-4.1875, 26.6255) (-4.2026, 26.647) (-4.2127, 26.6614) (-4.2178, 26.6685) knots 0 0 0 0 0 0 0.01428571 0.02857143 0.04285714 0.05714286 0.07142857 0.08571429 0.1 0.11428571 0.12857143 0.14285714 0.15714286 0.17142857 0.18571429 0.2 0.21428571 0.22857143 0.24285714 0.25714286 0.27142857 0.28571429 0.3 0.31428571 0.32857143 0.34285714 0.35714286 0.37142857 0.38571429 0.4 0.41428571 0.42857143 0.44285714 0.45714286 0.47142857 0.48571429 0.5 0.51428571 0.52857143 0.54285714 0.55714286 0.57142857 0.58571429 0.6 0.61428571 0.62857143 0.64285714 0.65714286 0.67142857 0.68571429 0.7 0.71428571 0.72857143 0.74285714 0.75714286 0.77142857 0.78571429 0.8 0.81428571 0.82857143 0.84285714 0.85714286 0.87142857 0.88571429 0.9 0.91428571 0.92857143 0.94285714 0.95714286 0.97142857 0.98571429 1 1 1 1 1 1
  arc A22 (-4.2178, 26.6685) -> (-5.8957, 26.3484) centre (0, 0) ccw